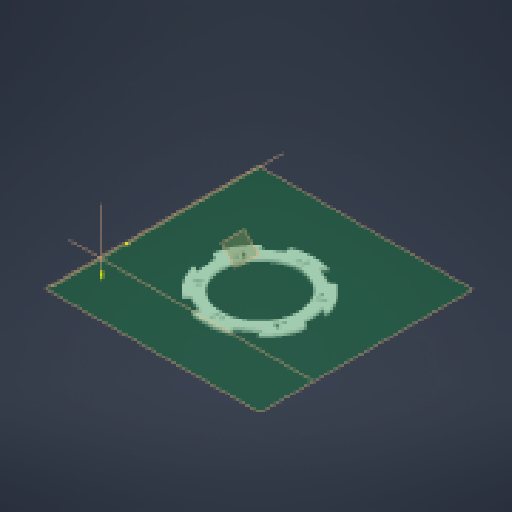
# Autodesk Inventor part: lower_centering_ring
Saved by Autodesk Inventor 2023 (Build 270158000, 158)
## iProperties
Created: 2022-06-17
Part Number: lower_centering_ring
Material: Generic
Document SubType Name: Modeling
Designer: bananenbrot
Density: 1 g/cm^3
Appearance: Default
Author: bananenbrot
Autodesk Inventor part; units mm, degrees
ref_plane "YZ Plane" through (0, 0, 0) normal (1, 0, 0) x (0, 1, 0)
ref_plane "XZ Plane" through (0, 0, 0) normal (0, 1, 0) x (-1, 0, 0)
ref_plane "XY Plane" through (0, 0, 0) normal (0, 0, 1) x (1, 0, 0)
ref_plane "Work Plane1" through (68.1481, 9.1828, -76.1575) normal (0.304, 0.3102, 0.9007) x (-0.7142, 0.6999, 0)
sketch "Sketch1" plane through (68.1481, 9.1828, -76.1575) normal (0.304, 0.3102, 0.9007) x (-0.7142, 0.6999, 0)
  point P0 (42.2443, 81.9528)
ref_plane "Work Plane2" through (96.1325, -13.384, -67.5182) normal (0, -1, 0) x (1, 0, 0)
sketch "Sketch2" plane through (96.1325, -13.384, -67.5182) normal (0, -1, 0) x (1, 0, 0)
  spline S0 degree 3 poles (52.1699, -11.7984) (52.8327, -11.5553) (53.4945, -11.3089) (54.7771, -10.8241) (55.3983, -10.5861) (56.0183, -10.3453) knots -0.420216 -0.420216 -0.420216 -0.420216 -0.208413 -0.208413 -0.008868 -0.008868 -0.008868 -0.008868
  spline S1 degree 3 poles (56.0183, -10.3453) (56.9856, -5.1078) (57.2145, 0.2452) (56.694, 5.5565) knots -30.680031 -30.680031 -30.680031 -30.680031 -29.077123 -29.077123 -29.077123 -29.077123
  spline S2 degree 3 poles (56.694, 5.5565) (56.6071, 5.52) (56.5202, 5.4836) (56.3142, 5.3974) (56.195, 5.3477) (56.0758, 5.298) knots -0.067003 -0.067003 -0.067003 -0.067003 -0.038747 -0.038747 0 0 0 0
  spline S3 degree 3 poles (56.0758, 5.298) (55.6471, 5.1131) (55.2178, 4.9295) (54.3549, 4.5635) (53.9213, 4.3811) (53.4871, 4.2001) knots -0.281176 -0.281176 -0.281176 -0.281176 -0.141113 -0.141113 0 0 0 0
  spline S4 degree 3 poles (53.4871, 4.2001) (53.434, 1.5454) (53.3027, -1.1109) (52.8701, -6.4471) (52.566, -9.1298) (52.1699, -11.7984) knots -1.606094 -1.606094 -1.606094 -1.606094 -0.809378 -0.809378 -0.00002 -0.00002 -0.00002 -0.00002
  spline S5 degree 3 poles (-36.3027, -39.2813) (-36.4236, -39.9768) (-36.541, -40.6731) (-36.7625, -42.0263) (-36.8669, -42.6833) (-36.9685, -43.3406) knots -0.420216 -0.420216 -0.420216 -0.420216 -0.208413 -0.208413 -0.008868 -0.008868 -0.008868 -0.008868
  spline S6 degree 3 poles (-36.9685, -43.3406) (-36.8003, -43.4841) (-36.6312, -43.6266) (-32.5277, -47.045) (-28.1784, -49.77) (-23.5349, -51.8766) knots -6.74235 -6.74235 -6.74235 -6.74235 -6.675988 -6.675988 -5.140113 -5.140113 -5.140113 -5.140113
  spline S7 degree 3 poles (-23.5349, -51.8766) (-23.5231, -51.7832) (-23.5112, -51.6898) (-23.4828, -51.4682) (-23.4663, -51.3401) (-23.4496, -51.2121) knots -0.067003 -0.067003 -0.067003 -0.067003 -0.038747 -0.038747 0 0 0 0
  spline S8 degree 3 poles (-23.4496, -51.2121) (-23.3955, -50.7483) (-23.3399, -50.2847) (-23.2254, -49.3545) (-23.1665, -48.8878) (-23.1061, -48.4213) knots -0.281176 -0.281176 -0.281176 -0.281176 -0.141113 -0.141113 0 0 0 0
  spline S9 degree 3 poles (-23.1061, -48.4213) (-25.3786, -47.0479) (-27.6134, -45.606) (-32.0185, -42.5633) (-34.1896, -40.9586) (-36.3027, -39.2813) knots -1.606094 -1.606094 -1.606094 -1.606094 -0.809378 -0.809378 -0.00002 -0.00002 -0.00002 -0.00002
  spline S10 degree 3 poles (-15.8672, 51.0797) (-16.4092, 51.5322) (-16.9535, 51.982) (-18.0146, 52.8504) (-18.5313, 53.2693) (-19.0498, 53.686) knots -0.420216 -0.420216 -0.420216 -0.420216 -0.208413 -0.208413 -0.008868 -0.008868 -0.008868 -0.008868
  spline S11 degree 3 poles (-19.0498, 53.686) (-21.8894, 52.6784) (-24.6509, 51.4448) (-29.3344, 48.8867) (-31.2883, 47.6593) (-33.159, 46.3202) knots -18.710643 -18.710643 -18.710643 -18.710643 -17.802634 -17.802634 -17.109649 -17.109649 -17.109649 -17.109649
  spline S12 degree 3 poles (-33.159, 46.3202) (-33.084, 46.2632) (-33.009, 46.2061) (-32.8314, 46.0708) (-32.7287, 45.9924) (-32.6261, 45.914) knots -0.067007 -0.067007 -0.067007 -0.067007 -0.038749 -0.038749 -0.000005 -0.000005 -0.000005 -0.000005
  spline S13 degree 3 poles (-32.6261, 45.914) (-32.2516, 45.6352) (-31.8779, 45.3553) (-31.1295, 44.791) (-30.7548, 44.5067) (-30.381, 44.2211) knots -0.281176 -0.281176 -0.281176 -0.281176 -0.141113 -0.141113 0 0 0 0
  spline S14 degree 3 poles (-30.381, 44.2211) (-28.0554, 45.5025) (-25.6892, 46.7169) (-20.8517, 49.0105) (-18.3764, 50.0884) (-15.8672, 51.0797) knots -1.606094 -1.606094 -1.606094 -1.606094 -0.809378 -0.809378 -0.00002 -0.00002 -0.00002 -0.00002
  spline S15 degree 3 poles (-21.1727, -52.8847) (-19.8408, -53.418) (-18.4872, -53.9015) (-11.5685, -56.0808) (-5.7963, -56.9656) (0, -56.9656) knots -4.882349 -4.882349 -4.882349 -4.882349 -4.450658 -4.450658 -2.706188 -2.706188 -2.706188 -2.706188
  spline S16 degree 3 poles (0, -56.9656) (1.5977, -56.9656) (3.1973, -56.8984) (12.1859, -56.1392) (19.3848, -54.0771) (25.9858, -50.6934) (29.7232, -48.7775) (33.2374, -46.4542) (39.6908, -41.0775) (42.6103, -38.0405) (49.6892, -28.8286) (53.0169, -22.1203) (55.1244, -14.3786) (55.2741, -13.7921) (55.4143, -13.2037) knots -2.706188 -2.706188 -2.706188 -2.706188 -2.225329 -2.225329 0 0 0 1.259962 1.259962 2.519925 2.519925 4.745254 4.745254 4.926958 4.926958 4.926958 4.926958
  spline S17 degree 3 poles (55.4143, -13.2037) (54.2723, -13.6212) (53.1265, -14.0297) (50.7387, -14.8582) (49.4948, -15.2771) (48.2477, -15.6833) knots -0.758273 -0.758273 -0.758273 -0.758273 -0.393544 -0.393544 -0.000079 -0.000079 -0.000079 -0.000079
  spline S18 degree 3 poles (48.2477, -15.6833) (48.9986, -12.1143) (49.5641, -8.5055) (50.3443, -1.3754) (50.5705, 2.1506) (50.6533, 5.6721) knots -2.150215 -2.150215 -2.150215 -2.150215 -1.056765 -1.056765 -0.000013 -0.000013 -0.000013 -0.000013
  spline S19 degree 3 poles (50.6533, 5.6721) (51.6506, 6.0789) (52.6454, 6.4936) (54.5554, 7.3061) (55.4721, 7.7033) (56.3859, 8.1062) knots -0.640702 -0.640702 -0.640702 -0.640702 -0.317567 -0.317567 -0.017995 -0.017995 -0.017995 -0.017995
  spline S20 degree 3 poles (56.3859, 8.1062) (55.383, 15.0822) (53.0937, 21.8151) (45.9904, 34.4236) (41.122, 40.1134) (29.4782, 49.3066) (22.8141, 52.7221) (8.5519, 56.8064) (1.09, 57.4362) (-9.6742, 56.2417) (-13.0172, 55.5623) (-16.2724, 54.592) knots -28.82013 -28.82013 -28.82013 -28.82013 -26.703951 -26.703951 -24.478622 -24.478622 -22.253292 -22.253292 -20.027963 -20.027963 -19.004195 -19.004195 -19.004195 -19.004195
  spline S21 degree 3 poles (-16.2724, 54.592) (-15.3398, 53.8118) (-14.4131, 53.0237) (-12.5018, 51.3701) (-11.517, 50.5023) (-10.5417, 49.6254) knots -0.758273 -0.758273 -0.758273 -0.758273 -0.393544 -0.393544 -0.000079 -0.000079 -0.000079 -0.000079
  spline S22 degree 3 poles (-10.5417, 49.6254) (-14.008, 48.4911) (-17.4161, 47.1766) (-23.981, 44.2871) (-27.1477, 42.72) (-30.2388, 41.031) knots -2.150215 -2.150215 -2.150215 -2.150215 -1.056765 -1.056765 -0.000013 -0.000013 -0.000013 -0.000013
  spline S23 degree 3 poles (-30.2388, 41.031) (-31.0898, 41.6912) (-31.9464, 42.3454) (-33.605, 43.5933) (-34.4074, 44.1886) (-35.2131, 44.7785) knots -0.640702 -0.640702 -0.640702 -0.640702 -0.317567 -0.317567 -0.017995 -0.017995 -0.017995 -0.017995
  spline S24 degree 3 poles (-35.2131, 44.7785) (-38.5369, 42.1647) (-41.5671, 39.1829) (-48.9155, 30.1227) (-52.4182, 23.504) (-56.6893, 9.2966) (-57.4169, 1.8437) (-55.9744, -12.9216) (-53.8181, -20.0927) (-47.4378, -32.1471) (-43.6502, -37.1247) (-39.1419, -41.3883) knots -16.851671 -16.851671 -16.851671 -16.851671 -15.577305 -15.577305 -13.351975 -13.351975 -11.126646 -11.126646 -8.901317 -8.901317 -7.035008 -7.035008 -7.035008 -7.035008
  spline S25 degree 3 poles (-39.1419, -41.3883) (-38.9325, -40.1906) (-38.7133, -38.994) (-38.2369, -36.5119) (-37.9777, -35.2252) (-37.706, -33.9421) knots -0.758273 -0.758273 -0.758273 -0.758273 -0.393544 -0.393544 -0.000079 -0.000079 -0.000079 -0.000079
  spline S26 degree 3 poles (-37.706, -33.9421) (-34.9906, -36.3769) (-32.1481, -38.671) (-26.3633, -42.9117) (-23.4228, -44.8706) (-20.4145, -46.7031) knots -2.150215 -2.150215 -2.150215 -2.150215 -1.056765 -1.056765 -0.000013 -0.000013 -0.000013 -0.000013
  spline S27 degree 3 poles (-20.4145, -46.7031) (-20.5608, -47.7702) (-20.699, -48.8391) (-20.9504, -50.8995) (-21.0648, -51.8919) (-21.1727, -52.8847) knots -0.640702 -0.640702 -0.640702 -0.640702 -0.317567 -0.317567 -0.017995 -0.017995 -0.017995 -0.017995
  spline S28 degree 3 poles (-37.7853, -41.4079) (-37.6627, -40.6577) (-37.5362, -39.908) (-37.2728, -38.3964) (-37.1357, -37.6342) (-36.9942, -36.873) knots -0.460315 -0.460315 -0.460315 -0.460315 -0.232268 -0.232268 0 0 0 0
  spline S29 degree 3 poles (-36.9942, -36.873) (-34.5898, -38.8875) (-32.1002, -40.8011) (-27.0516, -44.382) (-24.4928, -46.0569) (-21.8838, -47.6392) knots -1.856033 -1.856033 -1.856033 -1.856033 -0.915385 -0.915385 0 0 0 0
  spline S30 degree 3 poles (-21.8838, -47.6392) (-21.9769, -48.3398) (-22.0666, -49.041) (-22.2383, -50.4359) (-22.3205, -51.1298) (-22.3995, -51.824) knots -0.42162 -0.42162 -0.42162 -0.42162 -0.209593 -0.209593 0 0 0 0
  spline S31 degree 3 poles (-22.3995, -51.824) (-22.4424, -52.1626) (-22.4847, -52.5014) (-22.5622, -53.1345) (-22.5977, -53.4289) (-22.6327, -53.7233) knots -0.204313 -0.204313 -0.204313 -0.204313 -0.101905 -0.101905 -0.01295 -0.01295 -0.01295 -0.01295
  spline S32 degree 3 poles (-22.6327, -53.7233) (-28.82, -51.1168) (-34.517, -47.458) (-45.0544, -37.7646) (-49.5839, -31.5832) (-56.0185, -17.8323) (-57.8621, -10.3941) (-58.5944, 4.7703) (-57.4761, 12.3515) (-52.3964, 26.6585) (-48.4836, 33.2476) (-40.9819, 41.6203) (-38.3015, 44.098) (-35.4152, 46.3055) knots -31.623011 -31.623011 -31.623011 -31.623011 -29.604974 -29.604974 -27.327668 -27.327668 -25.050362 -25.050362 -22.773057 -22.773057 -20.495751 -20.495751 -19.400518 -19.400518 -19.400518 -19.400518
  spline S33 degree 3 poles (-35.4152, 46.3055) (-34.58, 45.6986) (-33.7487, 45.0864) (-32.0438, 43.8128) (-31.1701, 43.1503) (-30.3019, 42.4815) knots -0.638388 -0.638388 -0.638388 -0.638388 -0.328754 -0.328754 0 0 0 0
  spline S34 degree 3 poles (-30.3019, 42.4815) (-27.5512, 43.9903) (-24.7419, 45.4041) (-18.9754, 48.0316) (-16.0122, 49.2432) (-13.0028, 50.3242) knots -1.90097 -1.90097 -1.90097 -1.90097 -0.959321 -0.959321 0 0 0 0
  spline S35 degree 3 poles (-13.0028, 50.3242) (-13.6243, 50.8695) (-14.2491, 51.4112) (-15.4919, 52.476) (-16.11, 52.9996) (-16.7307, 53.5198) knots -0.490981 -0.490981 -0.490981 -0.490981 -0.242951 -0.242951 0 0 0 0
  spline S36 degree 3 poles (-16.7307, 53.5198) (-16.7702, 53.5043) (-16.8097, 53.4889) (-16.8887, 53.458) (-16.9282, 53.4425) (-16.9676, 53.427) knots -0.025446 -0.025446 -0.025446 -0.025446 -0.012721 -0.012721 0 0 0 0
  spline S37 degree 3 poles (-16.9676, 53.427) (-16.3792, 52.9457) (-15.7932, 52.4613) (-14.6158, 51.4774) (-14.0243, 50.9775) (-13.4358, 50.4745) knots -0.460315 -0.460315 -0.460315 -0.460315 -0.232268 -0.232268 0 0 0 0
  spline S38 degree 3 poles (-13.4358, 50.4745) (-16.3827, 49.3994) (-19.2847, 48.2002) (-24.9102, 45.6184) (-27.64, 44.2398) (-30.3149, 42.7715) knots -1.856033 -1.856033 -1.856033 -1.856033 -0.915385 -0.915385 0 0 0 0
  spline S39 degree 3 poles (-30.3149, 42.7715) (-30.875, 43.2024) (-31.4375, 43.6307) (-32.5596, 44.4769) (-33.1195, 44.895) (-33.6812, 45.3105) knots -0.42162 -0.42162 -0.42162 -0.42162 -0.209593 -0.209593 0 0 0 0
  spline S40 degree 3 poles (-33.6812, 45.3105) (-33.9529, 45.517) (-34.2252, 45.723) (-34.7347, 46.1067) (-34.9719, 46.2847) (-35.2094, 46.4622) knots -0.204313 -0.204313 -0.204313 -0.204313 -0.101905 -0.101905 -0.01295 -0.01295 -0.01295 -0.01295
  spline S41 degree 3 poles (-35.2094, 46.4622) (-32.1525, 48.7787) (-28.8671, 50.7935) (-18.5658, 55.7797) (-11.1525, 57.7207) (4.001, 58.652) (11.5962, 57.6332) (25.9687, 52.7417) (32.6085, 48.9157) (44.0478, 38.9339) (48.738, 32.8736) (55.054, 20.25) (56.9699, 13.973) (57.8093, 7.5178) knots -19.374528 -19.374528 -19.374528 -19.374528 -18.218445 -18.218445 -15.94114 -15.94114 -13.663834 -13.663834 -11.386528 -11.386528 -9.109223 -9.109223 -7.151877 -7.151877 -7.151877 -7.151877
  spline S42 degree 3 poles (57.8093, 7.5178) (56.8662, 7.0979) (55.9203, 6.6841) (53.9649, 5.8444) (52.9543, 5.4189) (51.941, 5.0015) knots -0.638388 -0.638388 -0.638388 -0.638388 -0.328754 -0.328754 0 0 0 0
  spline S43 degree 3 poles (51.941, 5.0015) (51.8723, 1.8648) (51.692, -1.2749) (51.0843, -7.5826) (50.6519, -10.7546) (50.0834, -13.9014) knots -1.90097 -1.90097 -1.90097 -1.90097 -0.959321 -0.959321 0 0 0 0
  spline S44 degree 3 poles (50.0834, -13.9014) (50.8664, -13.6358) (51.6479, -13.3655) (53.1915, -12.8216) (53.954, -12.5482) (54.7148, -12.2707) knots -0.490981 -0.490981 -0.490981 -0.490981 -0.242951 -0.242951 0 0 0 0
  spline S45 degree 3 poles (54.7148, -12.2707) (54.7212, -12.2287) (54.7276, -12.1868) (54.7403, -12.1029) (54.7467, -12.061) (54.753, -12.0191) knots -0.025446 -0.025446 -0.025446 -0.025446 -0.012721 -0.012721 0 0 0 0
  spline S46 degree 3 poles (54.753, -12.0191) (54.042, -12.288) (53.3294, -12.5533) (51.8886, -13.081) (51.16, -13.3433) (50.4301, -13.6014) knots -0.460315 -0.460315 -0.460315 -0.460315 -0.232268 -0.232268 0 0 0 0
  spline S47 degree 3 poles (50.4301, -13.6014) (50.9725, -10.5119) (51.3849, -7.399) (51.9618, -1.2363) (52.1328, 1.8171) (52.1987, 4.8677) knots -1.856033 -1.856033 -1.856033 -1.856033 -0.915385 -0.915385 0 0 0 0
  spline S48 degree 3 poles (52.1987, 4.8677) (52.8519, 5.1374) (53.5041, 5.4103) (54.7979, 5.959) (55.44, 6.2348) (56.0806, 6.5135) knots -0.42162 -0.42162 -0.42162 -0.42162 -0.209593 -0.209593 0 0 0 0
  spline S49 degree 3 poles (56.0806, 6.5135) (56.3954, 6.6456) (56.7099, 6.7784) (57.297, 7.0278) (57.5697, 7.1442) (57.8421, 7.2612) knots -0.204313 -0.204313 -0.204313 -0.204313 -0.101905 -0.101905 -0.01295 -0.01295 -0.01295 -0.01295
  spline S50 degree 3 poles (57.8421, 7.2612) (57.964, 6.2908) (58.0615, 5.3164) (58.6994, -3.231) (57.7804, -10.8389) (53.078, -25.2743) (49.3394, -31.9638) (39.5086, -43.5331) (33.5103, -48.3024) (26.7668, -51.7878) (22.9487, -53.7612) (18.924, -55.3064) (10.6083, -57.4837) (6.3429, -58.1092) (1.3648, -58.2841) (0.6821, -58.2961) (0, -58.2961) knots -7.125952 -7.125952 -7.125952 -7.125952 -6.831917 -6.831917 -4.554611 -4.554611 -2.277306 -2.277306 0 0 0 1.289391 1.289391 2.578782 2.578782 2.783744 2.783744 2.783744 2.783744
  spline S51 degree 3 poles (0, -58.2961) (-6.8971, -58.2961) (-13.7454, -57.072) (-20.9538, -54.4057) (-21.6772, -54.1215) (-22.3941, -53.8232) knots -33.954623 -33.954623 -33.954623 -33.954623 -31.882279 -31.882279 -31.648926 -31.648926 -31.648926 -31.648926
  spline S52 degree 3 poles (-22.3941, -53.8232) (-22.2862, -52.7965) (-22.1716, -51.7704) (-21.9211, -49.6572) (-21.7842, -48.5692) (-21.6391, -47.483) knots -0.638388 -0.638388 -0.638388 -0.638388 -0.328754 -0.328754 0 0 0 0
  spline S53 degree 3 poles (-21.6391, -47.483) (-24.3212, -45.8552) (-26.9501, -44.1291) (-32.1089, -40.449) (-34.6397, -38.4886) (-37.0807, -36.4229) knots -1.90097 -1.90097 -1.90097 -1.90097 -0.959321 -0.959321 0 0 0 0
  spline S54 degree 3 poles (-37.0807, -36.4229) (-37.2421, -37.2337) (-37.3988, -38.0457) (-37.6996, -39.6544) (-37.844, -40.4515) (-37.9841, -41.2491) knots -0.490981 -0.490981 -0.490981 -0.490981 -0.242951 -0.242951 0 0 0 0
  spline S55 degree 3 poles (-37.9841, -41.2491) (-37.951, -41.2756) (-37.9179, -41.3021) (-37.8516, -41.355) (-37.8185, -41.3815) (-37.7853, -41.4079) knots -0.025446 -0.025446 -0.025446 -0.025446 -0.012721 -0.012721 0 0 0 0
  circle A0 centre (0, 0) radius 39.5938
  line L0 (1.5, -67.0053) -> (1.5, -71.1884) projected
  line L1 (0, -140) -> (0, 140)
  line L2 (140.2771, 0) -> (-141.6627, 0)
  line L3 (43.0253, 26.5727) -> (44.5253, 23.9746) projected
  line L4 (37.5971, 19.9746) -> (44.5253, 23.9746) projected
  line L5 (37.5971, 19.9746) -> (36.0971, 22.5727) projected
  line L6 (43.0253, 26.5727) -> (36.0971, 22.5727) projected
  line L7 (-44.5253, 23.9746) -> (-43.0253, 26.5727) projected
  line L8 (-36.0971, 22.5727) -> (-43.0253, 26.5727) projected
  line L9 (-36.0971, 22.5727) -> (-37.5971, 19.9746) projected
  line L10 (-44.5253, 23.9746) -> (-37.5971, 19.9746) projected
  line L11 (1.5, -50.5474) -> (-1.5, -50.5474) projected
  line L12 (-1.5, -42.5474) -> (-1.5, -50.5474) projected
  line L13 (-1.5, -42.5474) -> (1.5, -42.5474) projected
  line L14 (1.5, -50.5474) -> (1.5, -42.5474) projected
  line L15 (33.5393, 21.096) -> (35.0393, 18.4979) projected
  ellipse E0 centre (14.6601, 96.7614) end of major axis (75.3021, 242.3405) minor radius 105.2986 (10.5417, -49.6254) -> (30.2388, -41.031) ccw projected
  ellipse E1 centre (101.9091, -55.2171) end of major axis (-17.3612, 3.3338) minor radius 45.663 (10.5417, -49.6254) -> (16.2724, -54.592) ccw projected
  ellipse E2 centre (73.1913, -40.8924) end of major axis (1.0809, 0.0011) minor radius 23.8597 (30.2388, -41.031) -> (35.2131, -44.7785) ccw projected
  ellipse E3 centre (76.4678, -61.0767) end of major axis (-19.2865, 64.2304) minor radius 105.2986 (-48.2477, 15.6833) -> (-50.6533, -5.6721) ccw projected
  ellipse E4 centre (-72.0095, -42.9393) end of major axis (-143.4796, -84.942) minor radius 23.8597 (-50.6533, -5.6721) -> (-56.3859, -8.1062) ccw projected
  ellipse E5 centre (-98.7739, -60.6473) end of major axis (-209.1157, -134.663) minor radius 45.663 (-48.2477, 15.6833) -> (-55.4143, 13.2037) ccw projected
  ellipse E6 centre (-91.1279, -35.6847) end of major axis (-247.5241, -55.9567) minor radius 105.2986 (37.706, 33.9421) -> (20.4145, 46.7031) ccw projected
  ellipse E7 centre (-3.1352, 115.8644) end of major axis (5.7934, -16.7022) minor radius 45.663 (37.706, 33.9421) -> (39.1419, 41.3883) ccw projected
  ellipse E8 centre (-1.1818, 83.8318) end of major axis (-1.8221, 166.728) minor radius 23.8597 (20.4145, 46.7031) -> (21.1727, 52.8847) ccw projected
  point P0 (-96.1325, 67.5182)
  point P1 (-55.4143, 13.2037)
  point P2 (-48.2477, 15.6833)
  point P3 (-50.6533, -5.6721)
  point P4 (-56.3859, -8.1062)
  point P5 (16.2723, -54.592)
  point P6 (10.5417, -49.6254)
  point P7 (30.2388, -41.031)
  point P8 (35.2131, -44.7785)
  point P9 (39.1419, 41.3883)
  point P10 (21.1727, 52.8847)
  constraints: 4 end point, 1 centre point, 1 coincident, 1 horizontal, 1 midpoint, 1 tangent, 1 vertical, 231 other
extrude "Extrusion1" add sketch "Sketch2" along normal blind 3 contours L2 A0 L1 S20 E8 E6 E7 S19 S18 | S18 S17 S16 E2 E0 E1 L1 L11 L14 L13 A0 L2 | S15 S27 S26 S25 S24 E4 E3 L2 A0 L1 L13 L12 L11 | L1 A0 L2 E3 E5 S24 S23 S22 S21 S20
sketch "Sketch3" plane through (96.1325, -13.384, -67.5182) normal (0, 1, 0) x (1, 0, 0)
  point P0 (-96.1325, -67.5182)
sketch "Sketch4" plane through (96.1325, -16.384, -67.5182) normal (0, -1, 0) x (1, 0, 0)
  circle A0 centre (-42.0116, -17.661) radius 3 projected
  circle A1 centre (-42.0116, -17.661) radius 3 projected
  circle A2 centre (-5.711, -45.2136) radius 3 projected
  circle A3 centre (36.3007, -27.5526) radius 3 projected
  circle A4 centre (42.0116, 17.661) radius 3 projected
  circle A5 centre (0, 0) radius 45 construction
  circle A6 centre (5.711, 45.2136) radius 3 projected
  circle A7 centre (-36.3007, 27.5526) radius 3 projected
  circle A8 centre (-5.711, -45.2136) radius 2.25
  circle A9 centre (-42.0116, -17.661) radius 2.25
  circle A10 centre (-36.3007, 27.5526) radius 2.25
  circle A11 centre (5.711, 45.2136) radius 2.25
  circle A12 centre (42.0116, 17.661) radius 2.25
  circle A13 centre (36.3007, -27.5526) radius 2.25
  point P0 (-96.1325, 67.5182)
  dimension "d3" = 6
  dimension "d4" = 4.5
  dimension "d5" = 4.5
  dimension "d6" = 4.5
  dimension "d7" = 4.5
  dimension "d8" = 4.5
  dimension "d9" = 4.5
  constraints: 6 centre point, 6 coincident
  measures "d3" diameter of A7
  measures "d4" diameter of A8
  measures "d5" diameter of A9
  measures "d6" diameter of A10
  measures "d7" diameter of A11
  measures "d8" diameter of A12
  measures "d9" diameter of A13
extrude "Extrusion2" cut sketch "Sketch4" against normal blind 10 contours A8 | A9 | A10 | A11 | A12 | A13
sketch "Sketch5" plane through (96.1325, -16.384, -67.5182) normal (0, -1, 0) x (1, 0, 0)
  point P0 (-96.1325, 67.5182)
sketch "Sketch6" plane through (96.1325, -13.384, -67.5182) normal (0, 1, 0) x (1, 0, 0)
  line L0 (35.7349, 22.3636) -> (37.2349, 19.7655) projected
  line L1 (44.8875, 24.1838) -> (37.2349, 19.7655) projected
  line L2 (44.8875, 24.1838) -> (43.3875, 26.7818) projected
  line L3 (35.7349, 22.3636) -> (43.3875, 26.7818) projected
  line L4 (1.5, -42.1292) -> (-1.5, -42.1292) projected
  line L5 (-1.5, -50.9656) -> (-1.5, -42.1292) projected
  line L6 (-1.5, -50.9656) -> (1.5, -50.9656) projected
  line L7 (1.5, -42.1292) -> (1.5, -50.9656) projected
  line L8 (-37.2349, 19.7655) -> (-35.7349, 22.3636) projected
  line L9 (-43.3875, 26.7818) -> (-35.7349, 22.3636) projected
  line L10 (-43.3875, 26.7818) -> (-44.8875, 24.1838) projected
  line L11 (-37.2349, 19.7655) -> (-44.8875, 24.1838) projected
  point P0 (-96.1325, -67.5182)
extrude "Extrusion3" cut sketch "Sketch6" against normal blind 10
body "Solid1"
